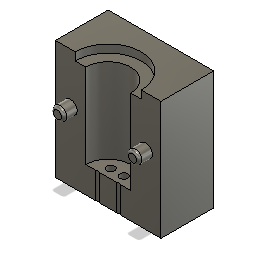
SaltLevelProbe v2 (Autodesk Fusion 360 design; units mm, degrees)
Autodesk Fusion 360 part; units mm, degrees
sketch "Sketch1" plane through (0, 0, 0) normal (0, 1, 0) x (1, 0, 0)
  circle A0 centre (0, 0) radius 8.5
  dimension "d2" = 17
  constraint coincident A0.centre origin
  measures "d2" diameter of A0
extrude "Extrude1" add sketch "Sketch1" along normal blind 2 makes body 1
sketch "Sketch3" plane through (0, 2, 0) normal (0, 1, 0) x (-1, 0, 0)
  circle A0 centre (0, 0) radius 8.5
  circle A1 centre (4.042, -1.3133) radius 1
  circle A2 centre (2.4981, 3.4383) radius 1
  circle A3 centre (-2.4981, 3.4383) radius 1
  circle A4 centre (-4.042, -1.3133) radius 1
  circle A5 centre (0, -4.25) radius 1
  dimension "d11" = 2
  dimension "d13" = 360
  measures "d11" diameter of A1
extrude "Extrude8" add 1 faces at (2.7075, 2, -1.6235) along direction (0, 1, 0) blind 30 on bodies 1 bodies 1
sketch "Sketch5" plane through (0, 32, 0) normal (0, 1, 0) x (-1, 0, 0)
  circle A0 centre (0, 0) radius 8.5
  circle A1 centre (0, 0) radius 12.5
  dimension "d28" = 25
  constraint concentric A0 A1
  measures "d28" diameter of A1
extrude "Extrude9" add sketch "Sketch5" along normal blind 3 contours A0 | A1 bodies 1
sketch "Sketch7" plane through (0, 35, 0) normal (0, 1, 0) x (-1, 0, 0)
  circle A0 centre (0, 0) radius 12.5
  line L0 (20, 20) -> (-20, 20)
  line L1 (-20, 20) -> (-20, -20)
  line L2 (-20, -20) -> (20, -20)
  line L3 (20, -20) -> (20, 20)
  line L4 (20, 20) -> (-20, -20) construction
  line L5 (-20, 20) -> (20, -20) construction
  dimension "d31" = 40
  dimension "d32" = 40
  constraint horizontal L0
  constraint perpendicular L0 L1
  constraint parallel L0 L2
  constraint parallel L1 L3
  constraint coincident L4 A0.centre
  constraint coincident L5 A0.centre
  constraint coincident A0.centre origin
  measures "d31" distance of L1.end L2.end
  measures "d32" distance of L0.end L1.end
extrude "Extrude1'" add sketch "Sketch7" against normal blind 45 separate body contours A0 | L0 L1 L2 L3 makes body 2 in component "Mold"
ref_plane "WorkPlane1" through (0, 12.5, 0) normal (0, 0, -1) x (1, 0, 0)
split "Split2" by plane through (0, 12.5, 0) normal (0, 0, -1) bodies 2 makes body 3 at (6.6667, 5, -20) in component "Mold"
mirror "Mirror1" about plane through (0, 12.5, 0) normal (0, 0, -1) of bodies 3 makes body 4 in component "Mold"
copy_body "Body->Comp1" bodies 4 removing the originals makes body 5 in component "MoldRight"
copy_body "Body->Comp2" bodies 3 removing the originals makes body 6 in component "MoldLeft"
sketch "Sketch8" plane through (0, 0, 0) normal (0, 0, 1) x (1, 0, 0)
  line L0 (-20, 35) -> (-20, -10)
  line L1 (-20, -10) -> (20, -10)
  line L2 (20, -10) -> (20, 35)
  line L3 (20, 35) -> (-20, 35)
  line L4 (-8.5, 16) -> (-20, 16) construction
  circle A0 centre (-14.25, 16) radius 2.5
  dimension "d37" = 5
  constraint coincident L0 L4.end
  constraint perpendicular L0 L4
  constraint midpoint L4 A0.centre
  measures "d37" diameter of A0
extrude "Extrude1''" add sketch "Sketch8" along normal blind 5 contours A0 bodies 6 in component "MoldLeft"
fillet "Fillet1" radius 1 1 edges at (-16.5808, 15.096, 5) on bodies 6 in component "MoldLeft"
sketch "Sketch9" plane through (0, 0, 0) normal (0, -1, 0) x (1, 0, 0)
  circle A0 centre (0, 0) radius 8.5
  line L0 (0, 0) -> (0, 4.25) construction
  circle A1 centre (0, 4.25) radius 1.5
  circle A2 centre (-4.042, 1.3133) radius 1.5
  circle A3 centre (-2.4981, -3.4383) radius 1.5
  circle A4 centre (2.4981, -3.4383) radius 1.5
  circle A5 centre (4.042, 1.3133) radius 1.5
  dimension "d44" = 4.25
  dimension "d45" = 3
  dimension "d47" = 360
  constraint coincident A0.centre L0.start
  constraint vertical L0
  constraint coincident L0.end A1.centre
  measures "d44" distance of A0.centre L0.end
  measures "d45" diameter of A1
extrude "Extrude10" add sketch "Sketch9" along normal blind 90 contours A1 | A2 | A3 | A4 | A5 bodies 1
ref_plane "WorkPlane2" through (0, 12.5, -10) normal (1, 0, 0) x (0, 0, 1)
mirror "Mirror1'" about plane through (0, 12.5, -10) normal (1, 0, 0) of "Extrude1''", "Fillet1" in component "MoldLeft"
combine "Combine1" operation cut target body 5 tool bodies 6 keep tools in component "MoldRight"
copy_body "Body->Comp7" bodies 1 removing the originals makes body 7 in component "Plug"
combine "Combine1'" operation cut target body 6 tool bodies 7 keep tools in component "MoldLeft"
combine "Combine2" operation cut target body 5 tool bodies 7 keep tools in component "MoldRight"
component "Mold" placed x (1, 0, 0) y (0, 1, 0) z (0, 0, 1) at (0, 0, 0)
component "Plug" placed x (1, 0, 0) y (0, 1, 0) z (0, 0, 1) at (0, 0, 0)
component "MoldRight" placed x (1, 0, 0) y (0, 1, 0) z (0, 0, 1) at (0, 0, 0) in component "Mold"
component "MoldLeft" placed x (1, 0, 0) y (0, 1, 0) z (0, 0, 1) at (0, 0, 0) in component "Mold"
equation "d44 = ( 8.5 / 2 ) * 1 mm"
named bodies: "Plug"
